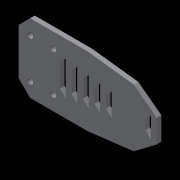
# Autodesk Inventor part: UpperArmMount
Saved by Autodesk Inventor 2020 (Build 240168000, 168)
## iProperties
Created: 2020-03-28
Part Number: UpperArmMount
Material: Generic
Document SubType Name: Modeling
Designer: valer
Density: 1 g/cm^3
Appearance: Default
Author: valer
Autodesk Inventor part; units mm, degrees
ref_plane "YZ Plane" through (0, 0, 0) normal (1, 0, 0) x (0, 1, 0)
ref_plane "XZ Plane" through (0, 0, 0) normal (0, 1, 0) x (-1, 0, 0)
ref_plane "XY Plane" through (0, 0, 0) normal (0, 0, 1) x (1, 0, 0)
sketch "Base" plane through (0, 0, 0) normal (0, 0, 1) x (1, 0, 0)
  line L0 (76.2, -12.7) -> (76.2, -19.05)
  line L1 (0, 0) -> (76.2, 0)
  line L2 (76.2, 0) -> (76.2, -76.2)
  line L3 (76.2, -76.2) -> (0, -76.2)
  line L4 (0, -76.2) -> (0, 0)
  line L5 (76.2, 0) -> (127, -6.2375)
  line L6 (127, -6.2375) -> (152.4, -25.3777)
  line L7 (152.4, -25.3777) -> (152.4, -38.1)
  line L8 (0, -38.1) -> (152.4, -38.1) construction
  line L9 (76.2, -76.2) -> (127, -69.9625)
  line L10 (127, -69.9625) -> (152.4, -50.8223)
  line L11 (152.4, -50.8223) -> (152.4, -38.1)
  circle A0 centre (12.7, -59.981) radius 3.175
  circle A1 centre (38.1, -59.981) radius 3.175
  circle A2 centre (38.1, -16.219) radius 3.175
  circle A3 centre (12.7, -16.219) radius 3.175
  line L12 (12.7, -59.981) -> (38.1, -59.981) construction
  line L13 (38.1, -59.981) -> (38.1, -16.219) construction
  line L14 (38.1, -16.219) -> (12.7, -16.219) construction
  line L15 (12.7, -16.219) -> (12.7, -59.981) construction
  circle A4 centre (12.7, -38.1) radius 3.175
  circle A5 centre (139.7, -38.1) radius 3.175
  point P0 (76.2, -38.1)
  dimension "d2" = 76.2
  dimension "d3" = 76.2
  dimension "d4" = 76.2
  dimension "d5" = 50.8
  dimension "d6" = 127
  dimension "d7" = 150
  dimension "d56" = 43.762
  dimension "d57" = 25.4
  dimension "d58" = 12.7
  dimension "d59" = 16.219
  dimension "d60" = 16.219
  dimension "d61" = 6.35
  dimension "d62" = 6.35
  dimension "d63" = 12.7
  constraints: 32 end point, 6 centre point, 4 midpoint, 4 parallel, 3 coincident, 3 symmetric about line, 2 horizontal, 2 perpendicular, 2 point on line, 1 vertical
  measures "d2" distance between parallel lines of L0 L4
  measures "d3" distance of L3.end L1.start
  measures "d4" distance from line of L2 L7.end
  measures "d5" horizontal distance of L1.end L5.end
  measures "d6" angle of L7 L6
  measures "d7" angle of L6 L5
  measures "d56" distance of L14.end L12.start
  measures "d57" distance of L12.start L12.end
  measures "d58" distance between parallel lines of L4 L15
  measures "d59" distance between parallel lines of L3 L12
  measures "d60" distance between parallel lines of L1 L14
  measures "d61" diameter of A4
  measures "d62" diameter of A5
  measures "d63" distance from line of L11 A5.centre
extrude "Extrusion1" add sketch "Base" along normal blind 5.08
chamfer "Chamfer1" distance 12.7 angle 45 2 edges at (0, 0, 2.54) (0, -76.2, 2.54)
sketch "Sketch5" plane through (0, 0, 0) normal (0, 0, -1) x (-1, 0, 0)
  line L0 (123.2486, -63.5) -> (-132.9007, -53.8026) construction
  line L1 (-132.9007, -22.3974) -> (123.2486, -12.7) construction
  line L2 (0, -12.7) -> (0, -63.5) projected
  line L3 (-96.323, -31.75) -> (-96.323, -44.45)
  line L4 (-96.323, -44.45) -> (-102.673, -50.8)
  line L5 (-102.673, -50.8) -> (-102.673, -25.4)
  line L6 (-102.673, -25.4) -> (-96.323, -31.75)
  line L7 (-45.523, -25.4) -> (-45.523, -50.8)
  line L8 (-45.523, -50.8) -> (-51.873, -57.15)
  line L9 (-51.873, -57.15) -> (-51.873, -19.05)
  line L10 (-51.873, -19.05) -> (-45.523, -25.4)
  line L11 (-58.223, -26.9875) -> (-58.223, -49.2125)
  line L12 (-58.223, -26.9875) -> (-64.573, -20.6375)
  line L13 (-64.573, -20.6375) -> (-64.573, -55.5625)
  line L14 (-64.573, -55.5625) -> (-58.223, -49.2125)
  line L15 (-51.873, -19.05) -> (-102.673, -25.4) construction
  line L16 (-51.873, -57.15) -> (-102.673, -50.8) construction
  line L17 (-77.273, -22.225) -> (-77.273, -53.975)
  line L18 (-77.273, -22.225) -> (-70.923, -28.575)
  line L19 (-70.923, -28.575) -> (-70.923, -47.625)
  line L20 (-70.923, -47.625) -> (-77.273, -53.975)
  line L21 (-89.973, -23.8125) -> (-89.973, -52.3875)
  line L22 (-89.973, -52.3875) -> (-83.623, -46.0375)
  line L23 (-83.623, -46.0375) -> (-83.623, -30.1625)
  line L24 (-83.623, -30.1625) -> (-89.973, -23.8125)
  point P0 (-45.523, -38.1)
  point P1 (-96.323, -38.1)
  point P2 (-58.223, -38.1)
  point P3 (-64.573, -38.1)
  point P4 (-89.973, -38.1)
  dimension "d34" = 45
  dimension "d35" = 6.35
  dimension "d37" = 38.1
  dimension "d39" = 45
  dimension "d40" = 6.35
  dimension "d41" = 25.4
  dimension "d42" = 6.35
  dimension "d43" = 6.35
  dimension "d44" = 6.35
  dimension "d45" = 6.35
  dimension "d46" = 6.35
  constraints: 44 end point, 9 parallel, 7 midpoint, 6 vertical, 2 perpendicular, 2 point on line
  measures "d34" angle of L8 L9
  measures "d35" distance between parallel lines of L9 L7
  measures "d37" distance of L8.end L9.end
  measures "d39" angle of L4 L5
  measures "d40" distance between parallel lines of L3 L5
  measures "d41" distance of L4.end L5.end
  measures "d42" distance between parallel lines of L9 L11
  measures "d43" distance between parallel lines of L13 L11
  measures "d44" distance between parallel lines of L19 L13
  measures "d45" distance between parallel lines of L23 L17
  measures "d46" distance between parallel lines of L3 L21
extrude "Extrusion2" cut sketch "Sketch5" against normal through all
equation "\"d60\" = d59"
equation "\"d34\" = d31"
equation "\"d35\" = d33"
equation "\"d39\" = d31"
equation "\"d40\" = d33"
equation "\"d42\" = d38"
equation "\"d43\" = d40"
equation "\"d44\" = d38"
equation "\"d45\" = d38"
equation "\"d46\" = d38"
equation "\"d31\" = 45deg"
equation "\"d33\" = 6.35"
equation "\"d38\" = 6.35"
body "Solid1"
